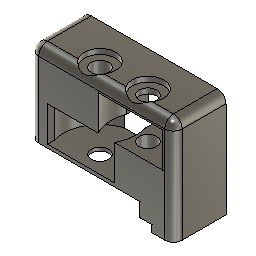
xOneFrame_SliderRollerHousing (Autodesk Fusion 360 design; units mm, degrees)
Autodesk Fusion 360 part; units mm, degrees
sketch "Skizze1" plane through (0, 0, 0) normal (0, 0, 1) x (1, 0, 0)
  circle A0 centre (0, 0) radius 9.5
  circle A1 centre (13.7, 0) radius 9.5
  circle A2 centre (13.7, 0) radius 2.5
  line L0 (12.9945, -5) -> (26, -5)
  line L1 (26, -5) -> (26, 10)
  line L2 (26, 10) -> (9.9945, 10)
  line L3 (9.9945, 10) -> (9.9945, -2)
  arc A3 (9.9945, -2) -> (12.9945, -5) centre (12.9945, -2) ccw
  line L4 (0.8934, -5) -> (-15, -5)
  line L5 (-15, -5) -> (-15, 10)
  line L6 (-15, 10) -> (3.8934, 10)
  line L7 (3.8934, 10) -> (3.8934, -2)
  arc A4 (0.8934, -5) -> (3.8934, -2) centre (0.8934, -2) ccw
  circle A5 centre (0, 0) radius 2.5
  line L8 (-10, 10) -> (-15, 10)
  line L9 (-15, 10) -> (-15, -5)
  line L10 (-15, -5) -> (-10, -5)
  line L11 (-10, -5) -> (-10, 10)
  circle A6 centre (0, 0) radius 10.4225
  line L12 (23.9945, 10) -> (23.9945, -5)
  circle A7 centre (13.7, 0) radius 10.5
  line L13 (14.85, 10) -> (14.85, -5)
  circle A8 centre (13.7, 0) radius 5.65
  line L14 (19.85, -5) -> (19.85, 10)
  line L15 (14.1927, -5) -> (9.1449, -5)
  line L16 (-0.5276, -5) -> (4.4669, -5)
  dimension "d1" = 19
  dimension "d2" = 19
  dimension "d3" = 13.7
  dimension "d4" = 5
  dimension "d5" = 3
  dimension "d8" = 3
  dimension "d9" = 5
  dimension "d12" = 21
  dimension "d18" = 15
  dimension "d19" = 26
  dimension "d22" = 1.15
  dimension "d23" = 11.3
  dimension "d26" = 5
  constraint coincident A0.centre A5.centre
  constraint concentric A1 A2
  constraint horizontal L0
  constraint vertical L1
  constraint horizontal L2
  constraint vertical L3
  constraint tangent L0 A3
  constraint tangent L3 A3
  constraint horizontal L4
  constraint vertical L5
  constraint horizontal L6
  constraint vertical L7
  constraint tangent L4 A4
  constraint tangent L7 A4
  constraint concentric A0 A5
  constraint horizontal L8
  constraint vertical L9
  constraint horizontal L10
  constraint vertical L11
  constraint coincident L6 L8.start
  constraint coincident L0 L12.end
  constraint perpendicular L0 L12
  constraint concentric A1 A7
  constraint coincident L2 L13.start
  constraint coincident L0 L13.end
  constraint perpendicular L0 L13
  constraint concentric A1 A8
  constraint coincident L0 L14.start
  constraint coincident L2 L14.end
  constraint perpendicular L2 L14
  constraint coincident L0 L15.start
  constraint coincident A6 L15.end
  constraint parallel L0 L15
  constraint coincident L4 L16.start
  constraint coincident A7 L16.end
  constraint parallel L4 L16
  measures "d1" diameter of A0
  measures "d2" diameter of A1
  measures "d3" distance of A0.centre A1.centre
  measures "d4" diameter of A2
  measures "d5" radius of A3
  measures "d8" radius of A4
  measures "d9" diameter of A5
  measures "d12" diameter of A7
  measures "d18" distance of L0.end L1.end
  measures "d19" distance of L1 A0.centre
  measures "d22" distance of A1.centre L13
  measures "d23" diameter of A8
  measures "d26" distance of L13 L14
extrude "Extrusion1" add sketch "Skizze1" against normal blind 11 contours A6 A8 L15 | A3 A6 A8 L15 | A2 L0 L3 A3 A6 L13 A8 L15 | A1 L3 L13 A8 | A1 L2 L3 A7 L13 | A2 L0 L13 A8 | A1 L0 L13 A8 L14 | A1 L0 L14 | A1 L0 L12 A7 L14 | L2 L3 A7 | A1 L2 A7 L13 L14 | L0 L12 A7 | L4 L5 L6 L8 L9 L10 L11 A6 | L0 L1 L2 L12 A7 | L12 A7 | L6 L11 A6 | L2 A7 L14 | L2 L12 A7 L14 makes body 1 at (22.6963, 1.9123, -11) makes body 2 at (-10.2339, -1.9736, -3.6667)
extrude "Extrusion2" add sketch "Skizze1" along normal blind 10 contours A0 L4 L7 A4 A7 L16 | A0 L4 L6 L7 L11 A6 | A4 A7 L16 | L6 L7 A6 | L4 L11 A6 | L0 L12 A7 | L4 L5 L6 L8 L9 L10 L11 A6 | L11 A6 | L0 L1 L2 L12 A7 | L6 L11 A6 | L2 A7 L14 | L2 L12 A7 L14 bodies 1 2
sketch "Skizze2" plane through (0, 0, 10) normal (0, 0, 1) x (-1, 0, 0)
  circle A0 centre (0, 0) radius 2.5
  line L0 (-3.8934, -10) -> (15, -10)
  line L1 (15, -10) -> (15, 5)
  line L2 (15, 5) -> (-4.4669, 5)
  line L3 (-3.8934, -3.7524) -> (-3.8934, -10)
  circle A1 centre (0, 0) radius 2.5
  circle A2 centre (-13.7, -0.0193) radius 2.5
  line L4 (15, -10) -> (-26, -10)
  line L5 (-26, -10) -> (-26, 5)
  line L6 (-26, 5) -> (15, 5)
  line L7 (15, 5) -> (15, -10)
  arc A3 (-3.8934, -3.7524) -> (-4.4669, 5) centre (-13.7, 0) ccw
  dimension "d13" = 5
  dimension "d14" = 5
  dimension "d15" = 13.7
  constraint coincident A0.centre A1.centre
  constraint horizontal L4
  constraint vertical L5
  constraint horizontal L6
  constraint vertical L7
  constraint coincident L0.end L1.start
  measures "d13" diameter of A1
  measures "d14" diameter of A2
  measures "d15" horizontal distance of A0.centre A2.centre
extrude "Extrusion3" add sketch "Skizze2" along normal blind 3 bodies 1 2
extrude "Extrusion4" add sketch "Skizze1" against normal blind 15 contours A1 L0 L13 A8 L14 | A1 L0 L14 | A1 L0 L12 A7 L14 | A1 L2 A7 L13 L14 | L0 L12 A7 | L0 L1 L2 L12 A7 | L12 A7 | L2 A7 L14 | L2 L12 A7 L14 bodies 1
extrude "Extrusion7" add sketch "Skizze1" against normal blind 17 contours A1 L0 L14 | A1 L0 L12 A7 L14 | L0 L12 A7 | L0 L1 L2 L12 A7 | L12 A7 | L2 L12 A7 L14 bodies 1
fillet "Abrundung1" radius 2.5 5 edges at (26, -5, 1) (5.5, -5, 13) (-15, -5, 1) (-15, 2.5, 13) (26, 2.5, 13) on bodies 1
sketch "Skizze3" plane through (0, 0, -11) normal (0, 0, -1) x (1, 0, 0)
  arc A0 (-12.5, 5) -> (-15, 2.5) centre (-12.5, 2.5) ccw
  line L0 (-15, 2.5) -> (-15, -10)
  line L1 (-15, -10) -> (-2.9374, -10)
  arc A1 (-10, 2.9374) -> (-2.9374, -10) centre (0, 0) ccw
  line L2 (-10, 2.9374) -> (-10, 5)
  line L3 (-10, 5) -> (-12.5, 5)
  line L4 (-12, 5) -> (13, 5)
  line L5 (13, 5) -> (13, -10)
  line L6 (13, -10) -> (-12, -10)
  line L7 (-12, -10) -> (-12, 5)
  circle A2 centre (13.7, 0) radius 2.5
  circle A3 centre (0, 0) radius 2.5
  line L8 (13, 5) -> (23, 5)
  line L9 (25.5, 2.5) -> (25.5, -10)
  line L10 (25.5, -10) -> (13, -10)
  line L11 (13, -10) -> (13, 5)
  arc A4 (25.5, 2.5) -> (23, 5) centre (23, 2.5) ccw
  dimension "d29" = 2.5
  constraint horizontal L4
  constraint vertical L5
  constraint horizontal L6
  constraint vertical L7
  constraint coincident L3 L4.start
  constraint coincident A1.centre A3.centre
  constraint horizontal L8
  constraint vertical L9
  constraint horizontal L10
  constraint vertical L11
  constraint tangent L8 A4
  constraint tangent L9 A4
  measures "d29" radius of A4
extrude "Extrusion5" add sketch "Skizze3" against normal blind 1 contours A1 L2 L4 L5 L6 A2 L11 bodies 1
sketch "Skizze4" plane through (0, 0, 13) normal (0, 0, 1) x (-1, 0, 0)
  line L0 (-23.5, 2.5) -> (-23.5, -10)
  line L1 (-23.5, -10) -> (12.5, -10)
  line L2 (12.5, -10) -> (12.5, 2.5)
  line L3 (12.5, 2.5) -> (0, 2.5)
  circle A0 centre (0, 0) radius 2.5
  line L4 (0, 2.5) -> (-23.5, 2.5)
  circle A1 centre (-13.7, -0.0193) radius 2.5
  circle A2 centre (0, 0) radius 4.5
  circle A3 centre (-13.7, -0.0193) radius 4.5
  dimension "d30" = 9
  dimension "d31" = 9
  constraint coincident A0.centre A2.centre
  constraint concentric A1 A3
  measures "d30" diameter of A2
  measures "d31" diameter of A3
extrude "Extrusion6" cut sketch "Skizze4" against normal blind 1.5 contours L4 A3 | L4 A3 | L3 L4 A2 | L3 L4 A2 bodies 1
equation "d23 = ( 5.65 * 2 ) * 1 mm"
